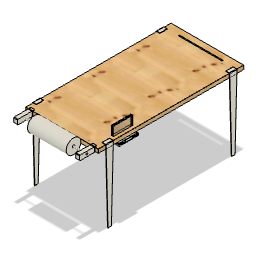
2024-04-11TrameTramTrame-setup (Autodesk Fusion 360 design; units mm, degrees)
Autodesk Fusion 360 part; units mm, degrees
note: some values were not read from the file. Chosen so that the rebuilt part matches the saved one: which bodies a step acts on.
sketch "Esquisse3" plane through (0, 0, 0) normal (0, 1, 0) x (1, 0, 0)
  line L0 (0, 0) -> (-750, 0)
  line L1 (-750, 0) -> (-750, 1500)
  line L2 (-750, 1500) -> (0, 1500)
  line L3 (0, 1500) -> (0, 0)
  dimension "d7" = 750
  dimension "d8" = 1500
  constraint horizontal L0
  constraint vertical L1
  constraint horizontal L2
  constraint vertical L3
  constraint coincident L0.start L3.end
  measures "d7" distance of L0.start L0.end
  measures "d8" distance of L0.start L2.end
extrude "Extrusion2" add sketch "Esquisse3" along normal blind 40 makes body 1
move_body "Déplacer1" bodies 1 to x (1, 0, 0) y (0, 1, 0) z (0, 0, 1) at (375, 750, 750)
move_body "Déplacer2" bodies 1 to x (1, 0, 0) y (0, 1, 0) z (0, 0, 1) at (0, -5, 0)
sketch "Esquisse4" plane through (0, 0, 0) normal (1, 0, 0) x (0, 0, -1)
  line L0 (461.292, 750) -> (536.292, 750)
  line L1 (536.292, 750) -> (516.292, 0)
  line L2 (536.292, 750) -> (461.292, 750)
  line L3 (481.292, 0) -> (461.292, 750)
  line L4 (516.292, 0) -> (481.292, 0)
  point P0 (498.792, 0)
  constraint horizontal L0
  constraint horizontal L4
move_body "Déplacer3" bodies 1 to x (1, 0, 0) y (0, 1, 0) z (0, 0, 1) at (0, -40, 0)
extrude "Extrusion3" add sketch "Esquisse4" along normal blind 5 separate body makes body 2
move_body "Déplacer4" bodies 2 to x (1, 0, 0) y (0, 1, 0) z (0, 0, 1) at (-380, 0, 0)
sketch "Esquisse5" plane through (0, 0, 0) normal (0, 1, 0) x (1, 0, 0)
  line L0 (0, 0) -> (40, 0)
  line L1 (40, 0) -> (40, 75)
  line L2 (40, 75) -> (0, 75)
  line L3 (0, 75) -> (0, 0)
  dimension "d16" = 40
  dimension "d17" = 75
  constraint horizontal L0
  constraint vertical L1
  constraint horizontal L2
  constraint vertical L3
  constraint coincident L0.start L3.end
  measures "d16" distance of L0.start L0.end
  measures "d17" distance of L0.start L2.end
extrude "Extrusion4" add sketch "Esquisse5" along normal blind 5 separate body makes body 3
move_body "Déplacer5" bodies 3 to x (1, 0, 0) y (0, 1, 0) z (0, 0, 1) at (-375, 750, -675)
move_body "Déplacer6" bodies 2 to x (1, 0, 0) y (0, 1, 0) z (0, 0, 1) at (0, 0, -213.708)
move_body "Déplacer7" bodies 3 to x (1, 0, 0) y (0, 1, 0) z (0, 0, 1) at (-5, 0, 0)
combine "Combiner1" operation add target body 3 tool bodies 2
copy_body "Copier/Coller des corps1" bodies 3 makes body 4
move_body "Déplacer8" bodies 4 to x (1, 0, 0) y (0, 1, 0) z (0, 0, 1) at (0, 0, 1425)
copy_body "Copier/Coller des corps2" bodies 3 4 makes body 5 makes body 6
move_body "Déplacer9" bodies 5 6 to x (1, 0, 0) y (0, 1, 0) z (0, 0, 1) at (750, 0, 0)
move_body "Déplacer10" bodies 6 to x (-1, 0, 0) y (0, 1, 0) z (0, 0, -1) at (750, 0, 1500)
move_body "Déplacer11" bodies 6 to x (1, 0, 0) y (0, 1, 0) z (0, 0, 1) at (0, 0, -75)
move_body "Déplacer12" bodies 5 to x (-1, 0, 0) y (0, 1, 0) z (0, 0, -1) at (750, 0, -1500)
move_body "Déplacer13" bodies 5 to x (1, 0, 0) y (0, 1, 0) z (0, 0, 1) at (0, 0, 75)
move_body "Déplacer14" bodies 1 to x (1, 0, 0) y (0, 1, 0) z (0, 0, 1) at (0, 5, 0)
move_body "Déplacer15" bodies 6 to x (1, 0, 0) y (0, 1, 0) z (0, 0, 1) at (0, 0, -75)
move_body "Déplacer16" bodies 5 to x (1, 0, 0) y (0, 1, 0) z (0, 0, 1) at (0, 0, 75)
move_body "Déplacer17" bodies 3 to x (1, 0, 0) y (0, 1, 0) z (0, 0, 1) at (0, 0, 75)
move_body "Déplacer18" bodies 4 to x (1, 0, 0) y (0, 1, 0) z (0, 0, 1) at (0, 0, -75)
sketch "Esquisse7" plane through (0, 0, 0) normal (0, 1, 0) x (1, 0, 0)
  line L0 (225, 675) -> (-225, 675)
  line L1 (-225, 675) -> (-225, 685)
  line L2 (-225, 685) -> (225, 685)
  line L3 (225, 685) -> (225, 675)
  dimension "d26" = 450
  dimension "d27" = 10
  constraint horizontal L0
  constraint perpendicular L0 L1
  constraint parallel L0 L2
  constraint parallel L1 L3
  measures "d26" distance of L1.end L2.end
  measures "d27" distance of L0.end L1.end
split "Scinder1" by curves path "Esquisse7" along L2 L3 L0 L1 bodies 1 makes body 7 at (75, 710, 275)
delete_body "RemoveBody1" bodies 1
sketch "Esquisse8" plane through (0, 750, 0) normal (0, 1, 0) x (-1, 0, 0)
  line L0 (225, -685) -> (-225, -685)
  line L1 (-225, -685) -> (-225, -675)
  line L2 (-225, -675) -> (225, -675)
  line L3 (225, -675) -> (225, -685)
  line L4 (-375, -750) -> (375, -750)
  line L5 (375, -750) -> (375, 750)
  line L6 (375, 750) -> (-375, 750)
  line L7 (-375, 750) -> (-375, -750)
  line L8 (-340, 560) -> (-330, 560)
  line L9 (-330, 560) -> (-330, 360)
  line L10 (-330, 360) -> (-340, 360)
  line L11 (-340, 360) -> (-340, 560)
  dimension "d30" = 10
  dimension "d31" = 200
  constraint horizontal L8
  constraint vertical L9
  constraint horizontal L10
  constraint vertical L11
  measures "d30" distance of L8.start L8.end
  measures "d31" distance of L8.start L10.end
split "Scinder2" by curves path "Esquisse8" along L11 L8 L9 L10 bodies 7 makes body 8 at (-90, 710, 145)
delete_body "RemoveBody2" bodies 7
fillet "Congé1" radius 5 1 edges at (380, 755, -637.5) on bodies 5
fillet "Congé2" radius 5 3 edges at (-380, 755, -637.5) (-380, 755, 637.5) (380, 755, 637.5) on bodies 3 4 6
fillet "Congé3" radius 1 1 faces at (125, 723.3333, 750) on bodies 8
fillet "Congé4" radius 1 10 faces at (-375, 723.3333, 249.3333) (-374.1269, 723.6667, 749.9919) (124.6667, 723.6667, 750) (-124.6667, 710.7412, 749.9659) (-90, 710, 144.6667) (374.1269, 723.6667, 749.9919) (375, 723.3333, -250.3333) (124.6667, 749.2588, 749.9659) (-90, 750, 144.6667) (-125, 723.3333, -750) on bodies 8
sketch "Esquisse9" plane through (0, 0, 0) normal (1, 0, 0) x (0, 0, -1)
  circle A0 centre (0, 0) radius 75
  dimension "d40" = 150
  constraint coincident A0.centre origin
  measures "d40" diameter of A0
extrude "Extrusion5" add sketch "Esquisse9" along normal blind 400 separate body makes body 9
move_body "Déplacer19" bodies 9 to x (1, 0, 0) y (0, 1, 0) z (0, 0, 1) at (-187.5, 0, 0)
move_body "Déplacer20" bodies 9 to x (1, 0, 0) y (0, 1, 0) z (0, 0, 1) at (0, 0, 850)
move_body "Déplacer21" bodies 9 to x (1, 0, 0) y (0, 1, 0) z (0, 0, 1) at (0, 650, -50)
hole "Perçage1" at (212.5, 650, 800) direction (-1, 0, 0) diameter 25 depth 400 tip angle 118 bodies 9
cylinder "CylindrePrimitive1" add diameter 20 height 680 placed x (0, 0, -1) y (0, 1, 0) z (1, 0, 0) at (0, 649.9213, 799.9829) separate body makes body 10
move_body "Déplacer22" bodies 10 to x (1, 0, 0) y (0, 1, 0) z (0, 0, 1) at (-340, 0, 0)
move_body "Déplacer23" bodies 9 to x (1, 0, 0) y (0, 1, 0) z (0, 0, 1) at (-10, 0, 0)
sketch "Esquisse11" plane through (0, 755, 0) normal (0, 1, 0) x (-1, 0, 0)
  line L0 (375, 600) -> (375, 675)
  line L1 (375, 675) -> (340, 675)
  line L2 (340, 675) -> (340, 600)
  line L3 (340, 600) -> (375, 600)
  line L4 (375, 675) -> (335, 675)
  line L5 (335, 675) -> (335, 700)
  line L6 (335, 700) -> (375, 700)
  line L7 (375, 700) -> (375, 675)
  dimension "d48" = 40
  dimension "d49" = 25
  constraint horizontal L4
  constraint vertical L5
  constraint horizontal L6
  constraint vertical L7
  constraint coincident L0.end L1.start
  measures "d48" distance of L0.end L4.end
  measures "d49" distance of L0.end L6.end
extrude "Extrusion6" add sketch "Esquisse11" along normal blind 5 separate body contours L1 L4 L5 L6 L7 makes body 11
move_body "Déplacer24" bodies 11 to x (1, 0, 0) y (0, 1, 0) z (0, 0, 1) at (0, 0, 55)
copy_body "Copier/Coller des corps3" bodies 11 makes body 12
move_body "Déplacer25" bodies 12 to x (1, 0, 0) y (0, 1, 0) z (0, 0, 1) at (750, 0, 0)
move_body "Déplacer26" bodies 12 to x (1, 0, 0) y (0, 1, 0) z (0, 0, 1) at (-40, 0, 0)
move_body "Déplacer27" bodies 11 to x (1, 0, 0) y (0, 1, 0) z (0, 0, 1) at (35, 0, 0)
move_body "Déplacer28" bodies 12 to x (1, 0, 0) y (0, 1, 0) z (0, 0, 1) at (-35, 0, 0)
move_body "Déplacer29" bodies 12 11 to x (1, 0, 0) y (0, 1, 0) z (0, 0, 1) at (0, -5, 0)
sketch "Esquisse12" plane through (0, 0, 0) normal (0, 0, 1) x (1, 0, 0)
  line L0 (0, 0) -> (40, 0)
  line L1 (40, 0) -> (40, -40)
  line L2 (40, -40) -> (0, -40)
  line L3 (0, -40) -> (0, 0)
  dimension "d52" = 40
  dimension "d53" = 40
  constraint horizontal L0
  constraint vertical L1
  constraint horizontal L2
  constraint vertical L3
  constraint coincident L0.start L3.end
  measures "d52" distance of L0.start L0.end
  measures "d53" distance of L0.start L2.end
extrude "Extrusion7" add sketch "Esquisse12" along normal blind 5 separate body makes body 13
move_body "Déplacer30" bodies 13 to x (1, 0, 0) y (0, 1, 0) z (0, 0, 1) at (-340, 0, 750)
copy_body "Copier/Coller des corps4" bodies 13 makes body 14
move_body "Déplacer31" bodies 14 to x (1, 0, 0) y (0, 1, 0) z (0, 0, 1) at (640, 0, 0)
move_body "Déplacer32" bodies 14 13 to x (1, 0, 0) y (0, 1, 0) z (0, 0, 1) at (0, 750, 0)
copy_body "Copier/Coller des corps5" bodies 11 12 makes body 15 makes body 16
move_body "Déplacer33" bodies 15 16 to x (1, 0, 0) y (0, 1, 0) z (0, 0, 1) at (0, -45, 0)
combine "Combiner2" operation add target body 13 tool bodies 11 15
combine "Combiner3" operation add target body 12 tool bodies 14 16
move_body "Déplacer34" bodies 10 9 to x (1, 0, 0) y (0, 1, 0) z (0, 0, 1) at (0, 0, 25)
move_body "Déplacer35" bodies 10 9 to x (1, 0, 0) y (0, 1, 0) z (0, 0, 1) at (0, -30, -70)
move_body "Déplacer36" bodies 10 9 to x (1, 0, 0) y (0, 1, 0) z (0, 0, 1) at (0, 0, -12)
sketch "Esquisse13" plane through (0, 0, 0) normal (0, 0, 1) x (1, 0, 0)
  line L0 (0, 0) -> (300, 0)
  line L1 (300, 705) -> (340, 705)
  line L2 (340, 705) -> (340, 590)
  line L3 (340, 590) -> (300, 590)
  line L4 (300, 590) -> (300, 705)
  dimension "d56" = 300
  dimension "d58" = 40
  dimension "d59" = 115
  constraint horizontal L0
  constraint coincident L0.start origin
  constraint horizontal L1
  constraint vertical L2
  constraint horizontal L3
  constraint vertical L4
  measures "d56" distance of L0.start L0.end
  measures "d58" distance of L1.start L1.end
  measures "d59" distance of L1.start L3.end
cylinder "CylindrePrimitive2" add diameter 10 height 10 placed x (1, 0, 0) y (0, 0, -1) z (0, 1, 0) at (-322.189, 755, 741.9157) separate body makes body 17
move_body "Déplacer39" bodies 17 to x (1, 0, 0) y (0, 1, 0) z (0, 0, 1) at (2, 0, 0)
cylinder "CylindrePrimitive3" add diameter 16.127 height 4 placed x (1, 0, 0) y (0, 0, -1) z (0, 1, 0) at (-320.189, 765, 741.9157) bodies 17
copy_body "Copier/Coller des corps7" bodies 17 makes body 18
move_body "Déplacer40" bodies 18 to x (1, 0, 0) y (0, 1, 0) z (0, 0, 1) at (641, 0, 0)
sketch "Esquisse16" plane through (0, 0, 0) normal (0, 0, 1) x (1, 0, 0)
sketch "Esquisse17" plane through (0, 750, 0) normal (0, 1, 0) x (-1, 0, 0)
  line L0 (-341, 359) -> (-341, 561)
  line L1 (-341, 561) -> (-329, 561)
  line L2 (-329, 561) -> (-329, 359)
  line L3 (-329, 359) -> (-341, 359)
  line L4 (-374, 749) -> (-374, -749)
  line L5 (-374, -749) -> (374, -749)
  line L6 (374, -749) -> (374, 749)
  line L7 (374, 749) -> (-374, 749)
  line L8 (226, -686) -> (-226, -686)
  line L9 (-226, -686) -> (-226, -674)
  line L10 (-226, -674) -> (226, -674)
  line L11 (226, -674) -> (226, -686)
  line L12 (-329, 359) -> (-341, 359)
  line L13 (-341, 359) -> (-341, 561)
  line L14 (-341, 561) -> (-329, 561)
  line L15 (-329, 561) -> (-329, 359)
  constraint horizontal L12
  constraint vertical L13
  constraint horizontal L14
  constraint vertical L15
  constraint coincident L0.end L1.start
  constraint coincident L2.end L3.start
extrude "Extrusion9" add sketch "Esquisse17" along normal blind 200 separate body contours L0 L1 L2 L3 L12 L13 L14 L15 makes body 19
move_body "Déplacer41" bodies 19 to x (1, 0, 0) y (0, 1, 0) z (0, 0, 1) at (0, -50, 0)
sketch "Esquisse18" plane through (0, 0, 0) normal (0, 1, 0) x (1, 0, 0)
  line L0 (341, -359) -> (411, -359)
  line L1 (411, -359) -> (411, -561)
  line L2 (411, -561) -> (341, -561)
  line L3 (341, -561) -> (341, -359)
  dimension "d72" = 70
  dimension "d73" = 202
  constraint horizontal L0
  constraint vertical L1
  constraint horizontal L2
  constraint vertical L3
  measures "d72" distance of L0.start L0.end
  measures "d73" distance of L0.start L2.end
extrude "Extrusion10" add sketch "Esquisse18" along normal blind 10 separate body makes body 20
move_face "DéplacerFace1" by (-80, 0, 0) 1 faces at (364.3333, 0, 426.3333) on bodies 20
move_body "Déplacer42" bodies 20 to x (1, 0, 0) y (0, 1, 0) z (0, 0, 1) at (-12, 0, 0)
move_body "Déplacer43" bodies 20 to x (1, 0, 0) y (0, 1, 0) z (0, 0, 1) at (0, 700, 0)
combine "Combiner4" operation add target body 19 tool bodies 20
move_body "Déplacer44" bodies 10 9 to x (1, 0, 0) y (0, 1, 0) z (0, 0, 1) at (0, 110, 90)
sketch "Esquisse20" plane through (0, 0, 0) normal (1, 0, 0) x (0, 0, -1)
  line L0 (0, 0) -> (-755, 0)
  line L1 (0, 755) -> (0, 0)
  line L2 (-755, 755) -> (-908, 755)
  line L3 (-908, 755) -> (-908, 705)
  line L4 (-908, 705) -> (-755, 705)
  line L5 (-755, 705) -> (-755, 755)
  dimension "d78" = 755
  dimension "d79" = 755
  dimension "d80" = 153
  dimension "d81" = 50
  constraint horizontal L0
  constraint vertical L1
  constraint coincident L0.start L1.end
  constraint horizontal L2
  constraint vertical L3
  constraint horizontal L4
  constraint vertical L5
  measures "d78" distance of L0.start L0.end
  measures "d79" distance of L0.start L1.start
  measures "d80" distance of L2.start L2.end
  measures "d81" distance of L2.start L4.end
extrude "Extrusion11" add sketch "Esquisse20" along normal blind 40 separate body makes body 21
move_body "Déplacer45" bodies 21 to x (1, 0, 0) y (0, 1, 0) z (0, 0, 1) at (300, 0, 0)
copy_body "Copier/Coller des corps8" bodies 21 makes body 22
move_body "Déplacer46" bodies 22 to x (1, 0, 0) y (0, 1, 0) z (0, 0, 1) at (-640, 0, 0)
move_body "Déplacer47" bodies 21 22 9 10 to x (1, 0, 0) y (0, 1, 0) z (0, 0, 1) at (0, 0, 20)
fillet "Congé5" radius 5 2 edges at (320, 755, 755) (320, 705, 755) on bodies 12
fillet "Congé6" radius 5 1 edges at (340, 752.5, 730) on bodies 12
fillet "Congé7" radius 5 1 edges at (300, 752.5, 730) on bodies 12
fillet "Congé8" radius 5 1 edges at (300, 707.5, 730) on bodies 12
fillet "Congé9" radius 5 1 edges at (340, 707.5, 730) on bodies 12
fillet "Congé10" radius 5 3 edges at (-340, 707.5, 730) (-300, 707.5, 730) (-320, 705, 755) on bodies 13
fillet "Congé11" radius 5 3 edges at (-300, 752.5, 730) (-320, 755, 755) (-340, 752.5, 730) on bodies 13
fillet "Congé12" radius 5 2 edges at (-320, 755, 775) (-320, 705, 775) on bodies 22
fillet "Congé13" radius 5 2 edges at (320, 755, 775) (320, 705, 775) on bodies 21
move_body "Déplacer48" bodies 9 22 21 10 to x (1, 0, 0) y (0, 1, 0) z (0, 0, 1) at (0, 0, -20)
fillet "Congé14" radius 5 4 edges at (320, 755, 908) (320, 705, 908) (-320, 755, 908) (-320, 705, 908) on bodies 21 22
sketch "Esquisse21" plane through (0, 0, 0) normal (0, 1, 0) x (1, 0, 0)
sketch "Esquisse24" plane through (0, 750, 0) normal (0, 1, 0) x (-1, 0, 0)
  line L0 (-341, 359) -> (-341, 561)
  line L1 (-341, 561) -> (-329, 561)
  line L2 (-329, 561) -> (-329, 359)
  line L3 (-329, 359) -> (-341, 359)
  line L4 (-374, 749) -> (-374, -749)
  line L5 (-374, -749) -> (374, -749)
  line L6 (374, -749) -> (374, 749)
  line L7 (374, 749) -> (-374, 749)
  line L8 (226, -686) -> (-226, -686)
  line L9 (-226, -686) -> (-226, -674)
  line L10 (-226, -674) -> (226, -674)
  line L11 (226, -674) -> (226, -686)
  line L12 (-340.0127, 360.0133) -> (-320.0127, 360.0133)
  line L13 (-320.0127, 360.0133) -> (-320.0127, 560.0133)
  line L14 (-320.0127, 560.0133) -> (-340.0127, 560.0133)
  line L15 (-340.0127, 560.0133) -> (-340.0127, 360.0133)
  dimension "d110" = 20
  dimension "d111" = 200
  constraint horizontal L12
  constraint vertical L13
  constraint horizontal L14
  constraint vertical L15
  measures "d110" distance of L12.start L12.end
  measures "d111" distance of L12.start L14.end
split "Scinder3" by curves path "Esquisse24" along L15 L12 L13 L14 bodies 8 makes body 23 at (-93.3291, 710, 145.0044)
delete_body "RemoveBody3" bodies 8
sketch "Esquisse25" plane through (0, 0, 0) normal (1, 0, 0) x (0, 0, -1)
  line L0 (0, 0) -> (-200, 0)
  line L1 (-200, 0) -> (-200, 250)
  line L2 (-200, 250) -> (0, 250)
  line L3 (0, 250) -> (0, 0)
  dimension "d112" = 200
  dimension "d113" = 250
  constraint horizontal L0
  constraint vertical L1
  constraint horizontal L2
  constraint vertical L3
  constraint coincident L0.start L3.end
  measures "d112" distance of L0.start L0.end
  measures "d113" distance of L0.start L2.end
extrude "Extrusion12" add sketch "Esquisse25" along normal blind 5 separate body makes body 24
sketch "Esquisse26" plane through (0, 0, 0) normal (0, 0, 1) x (1, 0, 0)
  line L0 (0, 0) -> (15, 0)
  line L1 (15, 0) -> (0.0039, 14.9961)
  line L2 (15, 0) -> (36.2077, 0) construction
  line L3 (0.0039, 14.9961) -> (0, 0)
  dimension "d116" = 15
  dimension "d117" = 135
  constraint coincident L0.start L3.end
  constraint horizontal L0
  constraint horizontal L2
  measures "d116" distance of L0.start L0.end
  measures "d117" angle of L1 L2
extrude "Extrusion13" add sketch "Esquisse26" along normal blind 200 separate body makes body 25
sketch "Esquisse27" plane through (0, 0, 0) normal (0, 0, 1) x (1, 0, 0)
  line L0 (0, 0) -> (80, 0)
  line L1 (80, 0) -> (80, 5)
  line L2 (80, 5) -> (0, 5)
  line L3 (0, 5) -> (0, 0)
  dimension "d120" = 80
  dimension "d121" = 5
  constraint horizontal L0
  constraint vertical L1
  constraint horizontal L2
  constraint vertical L3
  constraint coincident L0.start L3.end
  measures "d120" distance of L0.start L0.end
  measures "d121" distance of L0.start L2.end
extrude "Extrusion14" add sketch "Esquisse27" along normal blind 200 separate body makes body 26
sketch "Esquisse28" plane through (0, 0, 0) normal (0, 0, 1) x (1, 0, 0)
  line L0 (0, 0) -> (14.5664, 14.5664)
  line L1 (0, 0) -> (-20.6, 0) construction
  line L2 (0, 23.8282) -> (15, 23.8282)
  line L3 (15, -0.0151) -> (15, 14.9849)
  line L4 (15, 14.9849) -> (20, 14.9849)
  line L5 (20, 14.9849) -> (20, 249.9849)
  line L6 (20, 249.9849) -> (15, 249.9849)
  line L7 (15, 249.9849) -> (15, 14.9849)
  dimension "d124" = 135
  dimension "d125" = 20.6
  dimension "d126" = 15
  dimension "d127" = 15
  dimension "d128" = 5
  dimension "d129" = 235
  constraint horizontal L1
  constraint coincident L0.start L1.start
  constraint parallel L1 L2
  constraint perpendicular L2 L3
  constraint horizontal L4
  constraint vertical L5
  constraint horizontal L6
  constraint vertical L7
  measures "d124" angle of L0 L1
  measures "d125" distance of L0.start L0.end
  measures "d126" distance of L2.start L2.end
  measures "d127" distance of L3.start L3.end
  measures "d128" distance of L3.end L4.end
  measures "d129" distance of L3.end L6.end
extrude "Extrusion15" add sketch "Esquisse28" along normal blind 200 separate body makes body 27
sketch "Esquisse29" plane through (0, 0, 0) normal (0, 0, 1) x (1, 0, 0)
  line L0 (15.0022, -0.0115) -> (13.5093, -0.0115)
  line L1 (13.5093, -0.0115) -> (13.5093, 14.9885)
  line L2 (13.5093, 14.9885) -> (15.0022, 14.9885)
  line L3 (15.0022, 14.9885) -> (15.0022, -0.0115)
  line L4 (15.0022, 14.9885) -> (80.0022, 14.9885)
  line L5 (80.0022, 14.9885) -> (80.0022, 19.9885)
  line L6 (80.0022, 19.9885) -> (15.0022, 19.9885)
  line L7 (15.0022, 19.9885) -> (15.0022, 14.9885)
  dimension "d132" = 15
  dimension "d133" = 65
  dimension "d134" = 5
  constraint horizontal L0
  constraint vertical L1
  constraint horizontal L2
  constraint vertical L3
  constraint horizontal L4
  constraint vertical L5
  constraint horizontal L6
  constraint vertical L7
  measures "d132" distance of L0.start L2.end
  measures "d133" distance of L2.end L4.end
  measures "d134" distance of L2.end L6.end
extrude "Extrusion16" add sketch "Esquisse29" along normal blind 200 separate body contours L4 L5 L6 L7 makes body 28
move_face "DéplacerFace2" by (0, -100, 0) 1 faces at (1.6667, 250, 133.3333) on bodies 24
move_face "DéplacerFace3" by (0, -100, 0) 1 faces at (18.3333, 249.9849, 66.6667) on bodies 27
sketch "Esquisse30" plane through (0, 0, 0) normal (0, 0, 1) x (1, 0, 0)
  line L0 (0, 0) -> (20, 0)
  line L1 (20, 0) -> (20, 150)
  line L2 (20, 150) -> (0, 150)
  line L3 (0, 150) -> (0, 0)
  line L4 (0, 0) -> (80, 0)
  line L5 (80, 0) -> (80, 20)
  line L6 (80, 20) -> (0, 20)
  line L7 (0, 20) -> (0, 0)
  dimension "d137" = 20
  dimension "d138" = 150
  dimension "d139" = 80
  dimension "d140" = 20
  constraint horizontal L0
  constraint vertical L1
  constraint horizontal L2
  constraint vertical L3
  constraint coincident L0.start L3.end
  constraint horizontal L4
  constraint vertical L5
  constraint horizontal L6
  constraint vertical L7
  measures "d137" distance of L0.start L0.end
  measures "d138" distance of L0.start L2.end
  measures "d139" distance of L0.start L4.end
  measures "d140" distance of L0.start L6.end
extrude "Extrusion17" add sketch "Esquisse30" along normal blind 5 separate body makes body 29
move_face "DéplacerFace4" by (-10, 0, 0) 1 faces at (80.0022, 16.6551, 66.6667) on bodies 28
copy_body "Copier/Coller des corps9" bodies 29 makes body 30
move_body "Déplacer49" bodies 30 to x (1, 0, 0) y (0, 1, 0) z (0, 0, 1) at (0, 0, 195)
sketch "Esquisse31" plane through (0, 0, 0) normal (1, 0, 0) x (0, 0, -1)
  line L0 (0, 0) -> (-200, 0)
  line L1 (-200, 0) -> (-200, 10)
  line L2 (-200, 10) -> (0, 10)
  line L3 (0, 10) -> (0, 0)
  dimension "d143" = 200
  dimension "d144" = 10
  constraint horizontal L0
  constraint vertical L1
  constraint horizontal L2
  constraint vertical L3
  constraint coincident L0.start L3.end
  measures "d143" distance of L0.start L0.end
  measures "d144" distance of L0.start L2.end
extrude "Extrusion18" add sketch "Esquisse31" along normal blind 5 separate body makes body 31
move_body "Déplacer50" bodies 31 to x (1, 0, 0) y (0, 1, 0) z (0, 0, 1) at (75, 0, 0)
sketch "Esquisse32" plane through (0, 0, 0) normal (1, 0, 0) x (0, 0, -1)
  line L0 (-74.9982, 0) -> (-124.9982, 0)
  line L1 (-124.9982, 0) -> (-124.9982, 10)
  line L2 (-124.9982, 10) -> (-74.9982, 10)
  line L3 (-74.9982, 10) -> (-74.9982, 0)
  dimension "d147" = 50
  dimension "d148" = 10
  measures "d147" distance of L0.start L0.end
  measures "d148" distance of L0.start L2.end
split "Scinder4" by curves path "Esquisse32" along L1 L2 L3 L0 bodies 31 makes body 32 at (75, 3.3333, 149.9988) makes body 33 at (75, 3.3333, 49.9988)
delete_body "RemoveBody4" bodies 31
combine "Combiner5" operation add target body 29 tool bodies 26 25 24 28 30 33 27 32
move_body "Déplacer51" bodies 29 to x (1, 0, 0) y (0, 1, 0) z (0, 0, 1) at (320, 690, 360)
sketch "Esquisse33" plane through (0, 0, 0) normal (0, 0, 1) x (1, 0, 0)
sketch "Esquisse34" plane through (0, 0, 0) normal (0, 0, 1) x (1, 0, 0)
sketch "Esquisse35" plane through (340, 0, 0) normal (1, 0, 0) x (0, 0, -1)
  line L0 (-555, 839.9849) -> (-555, 840)
  line L1 (-555, 840) -> (-560, 840)
  line L2 (-560, 840) -> (-560, 710)
  line L3 (-560, 710) -> (-555, 710)
  line L4 (-555, 710) -> (-555, 709.9885)
  line L5 (-555, 709.9885) -> (-365, 709.9885)
  line L6 (-365, 709.9885) -> (-365, 710)
  line L7 (-365, 710) -> (-360, 710)
  line L8 (-360, 710) -> (-360, 840)
  line L9 (-360, 840) -> (-365, 840)
  line L10 (-365, 840) -> (-365, 839.9849)
  line L11 (-365, 839.9849) -> (-555, 839.9849)
hidden bodies 19
named bodies: "table", "pieda", "pieds", "pieds1", "pieds (1)", "pieds (1) (1)", "pieds2", "pieds3", "papier", "axe Rouleau", "Bracket R", "Bracket L", "visL", "visR", "distributeur", "protèse R", "protèse L", "table (1)", "distributeur v2"
